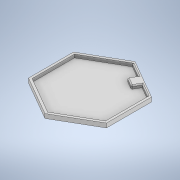
# Autodesk Inventor part: hexlight-bottom-led-module
Saved by Autodesk Inventor 2020 (Build 240168000, 168)
## iProperties
Created: 2019-10-02
Part Number: hexlight-bottom-led-module
Material: Generic
Document SubType Name: Modeling
Designer: Adam
Density: 1 g/cm^3
Appearance: Default
Author: Adam
Autodesk Inventor part; units mm, degrees
ref_plane "YZ Plane" through (0, 0, 0) normal (1, 0, 0) x (0, 1, 0)
ref_plane "XZ Plane" through (0, 0, 0) normal (0, 1, 0) x (-1, 0, 0)
ref_plane "XY Plane" through (0, 0, 0) normal (0, 0, 1) x (1, 0, 0)
sketch "Sketch1" plane through (0, 0, 0) normal (0, 1, 0) x (-1, 0, 0)
  line L0 (73.6122, 42.5) -> (73.6122, -42.5)
  line L1 (73.6122, -42.5) -> (0, -85)
  line L2 (0, -85) -> (-73.6122, -42.5)
  line L3 (-73.6122, -42.5) -> (-73.6122, 42.5)
  line L4 (-73.6122, 42.5) -> (0, 85)
  line L5 (0, 85) -> (73.6122, 42.5)
  point P0 (0, 0)
  point P1 (0, 0)
  dimension "d1" = 0
  dimension "d2" = 85
  constraints: 12 end point, 1 coincident, 13 other
  measures "d1" horizontal distance of point (0, 0) L4.end
  measures "d2" distance of L0.start L0.end
extrude "Extrusion1" add sketch "Sketch1" along normal blind 8
sketch "Sketch2" plane through (0, 8, 0) normal (0, 1, 0) x (1, 0, 0)
  line L0 (-69.282, -40) -> (-69.282, 40)
  line L1 (-69.282, 40) -> (0, 80)
  line L2 (0, 80) -> (69.282, 40)
  line L3 (69.282, 40) -> (69.282, -40)
  line L4 (69.282, -40) -> (0, -80)
  line L5 (0, -80) -> (-69.282, -40)
  point P0 (0, 0)
  point P1 (0, 0)
  dimension "d5" = 0
  dimension "d6" = 80
  constraints: 12 end point, 1 coincident, 13 other
  measures "d5" horizontal distance of point (0, 0) L4.end
  measures "d6" distance of L0.start L0.end
extrude "Extrusion2" cut sketch "Sketch2" against normal blind 6
sketch "Sketch4" plane through (0, 2, -80) normal (-0.5, 0, 0.8660254) x (0.8660254, 0, 0.5)
  line L0 (30, 6) -> (50, 6)
  line L1 (50, 6) -> (50, 0)
  line L2 (50, 0) -> (30, 0)
  line L3 (30, 0) -> (30, 6)
  line L4 (0, 0) -> (80, 0) projected
  line L5 (80, 6) -> (80, 0) projected
  line L6 (82.5, -2) -> (82.5, 6) projected
  point P0 (40, -2)
  dimension "d23" = 0
  dimension "d25" = 32.5
  dimension "d26" = 20
  dimension "d27" = 6
  constraints: 8 end point, 2 parallel, 1 horizontal, 1 perpendicular
  measures "d23" distance between parallel lines of L4 L2
  measures "d25" distance between parallel lines of L6 L1
  measures "d26" distance of L0.start L0.end
  measures "d27" distance of L0.end L1.end
extrude "Extrusion3" add sketch "Sketch4" along normal blind 15
fillet "Fillet1" radius 2 5 edges at (22.2308, 8, -58.5048) (12.9904, 8, -72.5) (39.5513, 8, -48.5048) (56.2917, 8, -47.5) (27.141, 8, -47.0096)
fillet "Fillet2" radius 2 4 edges at (19.281, 7.4142, -52.224) (18.4808, 4, -52.0096) (35.5869, 7.4142, -42.8098) (35.8013, 4, -42.0096)
body "Solid1"
